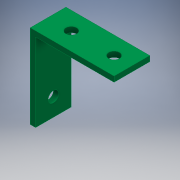
# Autodesk Inventor part: equerre_basse
Saved by Autodesk Inventor 2017 (Build 210142000, 142)
## iProperties
Created: 2017-04-14
Part Number: equerre_basse
Material: Generic
Document SubType Name: Modeling
Designer: franc
Density: 1 g/cm^3
Appearance: Default
Author: franc
Autodesk Inventor part; units mm, degrees
ref_plane "YZ Plane" through (0, 0, 0) normal (1, 0, 0) x (0, 1, 0)
ref_plane "XZ Plane" through (0, 0, 0) normal (0, 1, 0) x (-1, 0, 0)
ref_plane "XY Plane" through (0, 0, 0) normal (0, 0, 1) x (1, 0, 0)
sketch "Sketch1" plane through (0, 0, 0) normal (0, 1, 0) x (-1, 0, 0)
  line L0 (-15.0305, 11.0939) -> (8.4695, 11.0939)
  line L1 (8.4695, 11.0939) -> (8.4695, -12.4061)
  line L2 (8.4695, -12.4061) -> (6.9695, -12.4061)
  line L3 (6.9695, -12.4061) -> (6.9695, 9.5939)
  line L4 (6.9695, 9.5939) -> (-15.0305, 9.5939)
  line L5 (-15.0305, 9.5939) -> (-15.0305, 11.0939)
  point P0 (0, 0)
  dimension "d0" = 23.5
  dimension "d1" = 23.5
  dimension "d2" = 1.5
  dimension "d3" = 1.5
  constraints: 12 end point, 5 perpendicular, 1 horizontal
  measures "d0" distance of L0.start L0.end
  measures "d1" distance of L0.end L1.end
  measures "d2" distance of L4.end L0.start
  measures "d3" distance of L1.end L2.end
extrude "Extrusion1" add sketch "Sketch1" along normal blind 10
sketch "Sketch2" plane through (15.0305, 0, 9.5939) normal (0, 0, -1) x (-1, 0, 0)
  circle A0 centre (5, 5) radius 1.5
  circle A1 centre (17, 5) radius 1.5
  line L0 (0, 10) -> (22, 10) projected
  line L1 (0, 0) -> (0, 10) projected
  line L2 (23.5, 0) -> (23.5, 10) projected
  point P0 (15.0305, 0)
  dimension "d6" = 3
  dimension "d7" = 3
  dimension "d8" = 5
  dimension "d9" = 5
  dimension "d10" = 5
  dimension "d11" = 6.5
  constraints: 2 centre point
  measures "d6" diameter of A0
  measures "d7" diameter of A1
  measures "d8" distance from line of L0 A0.centre
  measures "d9" distance from line of L0 A1.centre
  measures "d10" distance from line of A0.centre L1
  measures "d11" distance from line of L2 A1.centre
extrude "Extrusion2" cut sketch "Sketch2" against normal up to next
sketch "Sketch3" plane through (-6.9695, 0, 9.5939) normal (1, 0, 0) x (0, 0, -1)
  circle A0 centre (17, 5) radius 1.5
  line L0 (0, 10) -> (22, 10) projected
  line L1 (-1.5, 0) -> (-1.5, 10) projected
  line L2 (22, 0) -> (22, 10) projected
  point P0 (9.5939, 0)
  dimension "d14" = 3
  dimension "d15" = 5
  dimension "d19" = 5
  constraints: 1 centre point
  measures "d14" diameter of A0
  measures "d15" distance from line of L0 A0.centre
  measures "d19" distance from line of L2 A0.centre
extrude "Extrusion3" cut sketch "Sketch3" against normal up to next
body "Solid1"
